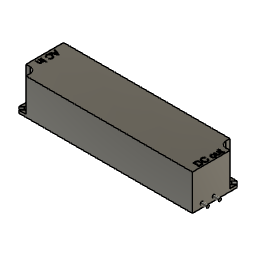
PSUBox (Autodesk Fusion 360 archive; units mm, degrees)
design "Meanwell LPV-35-5"
Autodesk Fusion 360 part; units mm, degrees
sketch "Base" plane through (0, 0, 0) normal (0, 0, 1) x (1, 0, 0) in component "Meanwell LPV-35-5"
  line L0 (0, 0) -> (148, 0)
  line L1 (148, 0) -> (148, 40)
  line L2 (148, 40) -> (0, 40)
  line L3 (0, 40) -> (0, 0)
  line L4 (144.5, 36.5) -> (3.5, 36.5) construction
  line L5 (3.5, 36.5) -> (3.5, 3.5) construction
  line L6 (3.5, 3.5) -> (144.5, 3.5) construction
  line L7 (144.5, 3.5) -> (144.5, 36.5) construction
  circle A0 centre (144.5, 36.5) radius 1.75
  circle A1 centre (148, 40) radius 1.75 construction
  line L8 (143.2626, 37.7374) -> (145.5251, 40)
  line L9 (145.7374, 35.2626) -> (148, 37.5251)
  circle A2 centre (3.5, 3.5) radius 1.75
  circle A3 centre (0, 0) radius 1.75 construction
  line L10 (4.7374, 2.2626) -> (2.4749, 0)
  line L11 (2.2626, 4.7374) -> (0, 2.4749)
  dimension "d1" = 148
  dimension "d2" = 40
  dimension "d3" = -3.5
  dimension "d5" = 3.5
  dimension "d6" = 3.5
  dimension "d7" = 3.5
  dimension "d8" = 3.5
  constraint horizontal L0
  constraint vertical L1
  constraint horizontal L2
  constraint vertical L3
  constraint coincident L0.start L3.end
  constraint coincident L4.start L7.end
  constraint coincident L1.end L2.start
  constraint coincident A0 L8.start
  constraint tangent A1 L8
  constraint tangent A0 L8
  constraint coincident A0 L9.start
  constraint tangent A1 L9
  constraint tangent A0 L9
  constraint coincident L2 L8.end
  constraint coincident L1 L9.end
  constraint coincident L5.end L6.start
  constraint coincident A2 L10.start
  constraint tangent A3 L10
  constraint coincident A2 L11.start
  constraint tangent A3 L11
  constraint tangent A2 L10
  constraint tangent A2 L11
  constraint coincident L0 L10.end
  constraint coincident L3 L11.end
  measures "d1" distance of L0.start L0.end
  measures "d2" distance of L0.start L2.end
  measures "d5" diameter of A0
  measures "d6" diameter of A1
  measures "d7" diameter of A2
  measures "d8" diameter of A3
extrude "Extrude1" add sketch "Base" along normal blind 2.22 contours L0 L1 L2 L3 A0 L8 L9 A2 L10 L11 in component "Meanwell LPV-35-5"
sketch "Body" plane through (0, 0, 2.22) normal (0, 0, 1) x (-1, 0, 0) in component "Meanwell LPV-35-5"
  line L0 (-4.7374, -2.2626) -> (-2.4749, 0)
  line L1 (-2.4749, 0) -> (-148, 0)
  line L2 (-148, 0) -> (-148, -37.5251)
  line L3 (-148, -37.5251) -> (-145.7374, -35.2626)
  arc A0 (-143.2626, -37.7374) -> (-145.7374, -35.2626) centre (-144.5, -36.5) ccw
  line L4 (-143.2626, -37.7374) -> (-145.5251, -40)
  line L5 (-145.5251, -40) -> (0, -40)
  line L6 (0, -40) -> (0, -2.4749)
  line L7 (0, -2.4749) -> (-2.2626, -4.7374)
  arc A1 (-4.7374, -2.2626) -> (-2.2626, -4.7374) centre (-3.5, -3.5) ccw
  line L8 (-139.5, -36.5) -> (-139.5, -40)
  line L9 (-144.5, -31.5) -> (-148, -31.5)
  arc A2 (-139.5, -36.5) -> (-144.5, -31.5) centre (-144.5, -36.5) ccw
  line L10 (-8.5, -3.5) -> (-8.5, 0)
  line L11 (-3.5, -8.5) -> (0, -8.5)
  arc A3 (-8.5, -3.5) -> (-3.5, -8.5) centre (-3.5, -3.5) ccw
  dimension "d11" = 10
  constraint concentric A0 A2
  constraint coincident L5 L8.end
  constraint tangent L8 A2
  constraint perpendicular L5 L8
  constraint coincident L2 L9.end
  constraint tangent L9 A2
  constraint perpendicular L2 L9
  constraint coincident L1 L10.end
  constraint perpendicular L1 L10
  constraint coincident L6 L11.end
  constraint perpendicular L6 L11
  measures "d11" diameter of A2
extrude "Extrude2" add sketch "Body" along normal blind 27.78 contours L1 L2 L5 L6 L8 L9 A2 L10 L11 A3 in component "Meanwell LPV-35-5"
sketch "DCout" plane through (148, 0, 0) normal (1, 0, 0) x (0, 1, 0) in component "Meanwell LPV-35-5"
  line L0 (0, 0) -> (37.5251, 0)
  line L1 (37.5251, 0) -> (37.5251, 2.22)
  line L2 (37.5251, 2.22) -> (31.5, 2.22)
  line L3 (31.5, 2.22) -> (31.5, 30)
  line L4 (31.5, 30) -> (0, 30)
  line L5 (0, 30) -> (0, 0)
  line L6 (0, 30) -> (18, 30) construction
  line L7 (18, 30) -> (18, 3.5) construction
  line L8 (18, 3.5) -> (0, 3.5) construction
  line L9 (0, 3.5) -> (0, 30) construction
  circle A0 centre (18, 3.5) radius 1.25
  line L10 (18, 3.5) -> (8, 3.5) construction
  circle A1 centre (8, 3.5) radius 1.25
  dimension "d15" = 18
  dimension "d16" = 26.5
  dimension "d17" = 2.5
  dimension "d20" = 10
  dimension "d21" = 2.5
  constraint horizontal L6
  constraint vertical L7
  constraint horizontal L8
  constraint vertical L9
  constraint coincident L4.end L5.start
  constraint coincident L7.end L8.start
  constraint perpendicular L7 L10
  constraint coincident L10.end A1.centre
  measures "d15" distance of L4.end L6.end
  measures "d16" distance of L4.end L8.end
  measures "d17" diameter of A0
  measures "d20" distance of L7.end L10.end
  measures "d21" diameter of A1
extrude "Extrude3" add sketch "DCout" along normal blind 5 contours A0 | A1 in component "Meanwell LPV-35-5"
sketch "ACinn" plane through (0, 0, 0) normal (-1, 0, 0) x (0, -1, 0) in component "Meanwell LPV-35-5"
  line L0 (-40, 0) -> (-2.4749, 0)
  line L1 (-2.4749, 0) -> (-2.4749, 2.22)
  line L2 (-2.4749, 2.22) -> (-8.5, 2.22)
  line L3 (-8.5, 2.22) -> (-8.5, 30)
  line L4 (-8.5, 30) -> (-40, 30)
  line L5 (-40, 30) -> (-40, 0)
  line L6 (-40, 30) -> (-22, 30) construction
  line L7 (-22, 30) -> (-22, 3.5) construction
  line L8 (-22, 3.5) -> (-40, 3.5) construction
  line L9 (-40, 3.5) -> (-40, 30) construction
  circle A0 centre (-22, 3.5) radius 1.25
  line L10 (-22, 3.5) -> (-32, 3.5) construction
  circle A1 centre (-32, 3.5) radius 1.25
  dimension "d22" = 18
  dimension "d23" = 26.5
  dimension "d24" = 2.5
  dimension "d25" = 10
  dimension "d26" = 2.5
  constraint horizontal L6
  constraint vertical L7
  constraint horizontal L8
  constraint vertical L9
  constraint coincident L4.end L5.start
  constraint coincident L7.end L8.start
  constraint perpendicular L7 L10
  constraint coincident L10.end A1.centre
  measures "d22" distance of L4.end L6.end
  measures "d23" distance of L4.end L8.end
  measures "d24" diameter of A0
  measures "d25" distance of L7.end L10.end
  measures "d26" diameter of A1
extrude "Extrude4" add sketch "ACinn" along normal blind 5 contours A0 | A1 in component "Meanwell LPV-35-5"
sketch "Sketch5" plane through (0, 0, 30) normal (0, 0, 1) x (-1, 0, 0) in component "Meanwell LPV-35-5"
  line L0 (-8.5, 0) -> (-148, 0)
  line L1 (-148, 0) -> (-148, -31.5)
  line L2 (-148, -31.5) -> (-144.5, -31.5)
  arc A0 (-139.5, -36.5) -> (-144.5, -31.5) centre (-144.5, -36.5) ccw
  line L3 (-139.5, -36.5) -> (-139.5, -40)
  line L4 (-139.5, -40) -> (0, -40)
  line L5 (0, -40) -> (0, -8.5)
  line L6 (0, -8.5) -> (-3.5, -8.5)
  arc A1 (-8.5, -3.5) -> (-3.5, -8.5) centre (-3.5, -3.5) ccw
  line L7 (-8.5, -3.5) -> (-8.5, 0)
  line L8 (-2.2058, -35) -> (-2.2058, -11) construction
  line L9 (-2.2058, -11) -> (-6.2058, -11) construction
  line L10 (-6.2058, -11) -> (-6.2058, -35) construction
  line L11 (-6.2058, -35) -> (-2.2058, -35) construction
  line L12 (-148, -5) -> (-148, -30) construction
  line L13 (-148, -30) -> (-140.3681, -30) construction
  line L14 (-140.3681, -30) -> (-140.3681, -5) construction
  line L15 (-140.3681, -5) -> (-148, -5) construction
  text T0 "AC in" font "Arial" height 5 align centre middle in box 24 x 4 at (-2.2058, -35) x (0, 1) y (-1, 0) spacing 1 kerned
  text T1 "DC out" font "Arial" height 5 align centre middle in box 25 x 7.6319 at (-148, -5) x (0, -1) y (1, 0) spacing 1 kerned
extrude "Extrude5" cut sketch "Sketch5" against normal blind 3 text T1 T0 in component "Meanwell LPV-35-5"
component "Meanwell LPV-35-5" placed x (1, 0, 0) y (0, 1, 0) z (0, 0, 1) at (0, 0, 0)
equation "d13 = 30 mm - 2.22 mm"
